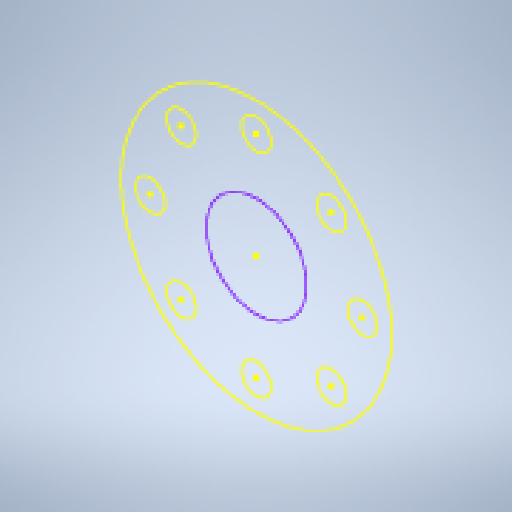
# Autodesk Inventor part: 부품69
Saved by Autodesk Inventor 2024 (Build 280153000, 153)
## iProperties
Created: 2024-09-08
Part Number: 부품69
Material: 일반
Document SubType Name: Modeling
Designer: Eungang
Density: 1 g/cm^3
Appearance: 기본값
Author: Eungang
Autodesk Inventor part; units mm, degrees
ref_plane "YZ Plane" through (0, 0, 0) normal (1, 0, 0) x (0, 1, 0)
ref_plane "XZ Plane" through (0, 0, 0) normal (0, 1, 0) x (-1, 0, 0)
ref_plane "XY Plane" through (0, 0, 0) normal (0, 0, 1) x (1, 0, 0)
sketch "스케치1" plane through (0, 0, 0) normal (0, 0, 1) x (1, 0, 0)
  circle A0 centre (-7.7782, -7.7782) radius 1.55 projected
  circle A1 centre (7.7782, -7.7782) radius 1.55 projected
  circle A2 centre (7.7782, 7.7782) radius 1.55 projected
  circle A3 centre (-7.7782, 7.7782) radius 1.55 projected
  circle A4 centre (0, 11) radius 1.55 projected
  circle A5 centre (11, 0) radius 1.55 projected
  circle A6 centre (0, -11) radius 1.55 projected
  circle A7 centre (-11, 0) radius 1.55 projected
  circle A8 centre (0, 0) radius 14 projected
  arc A9 (0, -5.2) -> (0, 5.2) centre (0, 0) ccw
  line L0 (32.5, -23) -> (32.5001, 127) projected
  line L1 (26.5, -23) -> (32.5, -23) projected
  line L2 (26.5001, 127) -> (26.5, -23) projected
  line L3 (32.5001, 127) -> (26.5001, 127) projected
  line L4 (0, 14) -> (32.5, 14)
  line L5 (32.5, 14) -> (32.5, -12.55)
  line L6 (0, -12.55) -> (0, 14)
  line L7 (0, -14) -> (32.5, -14)
  line L8 (32.5, -14) -> (32.5, -12.55)
  line L9 (0, 5.2) -> (-9.6, 5.2)
  line L10 (-9.6, -5.2) -> (0, -5.2)
  line L11 (0, -5.2) -> (0, 5.2)
  arc A10 (-11.2, -8.4) -> (-11.2, 8.4) centre (0, 0) ccw
  arc A11 (-11.2, 8.4) -> (-9.6, 5.2) centre (-9.6, 7.2) ccw
  arc A12 (-9.6, -5.2) -> (-11.2, -8.4) centre (-9.6, -7.2) ccw
  line L12 (26.5, 0) -> (32.5, 0)
  line L13 (32.5, 0) -> (32.5, -3)
  line L14 (32.5, -3) -> (26.5, -3)
  line L15 (26.5, -3) -> (26.5, 0)
  line L16 (32.5, 0) -> (26.5, 0)
  line L17 (26.5, 0) -> (26.5, 3)
  line L18 (26.5, 3) -> (32.5, 3)
  line L19 (32.5, 3) -> (32.5, 0)
  point P0 (0, 0)
  point P1 (-12.9985, -5.2)
  point P2 (-12.9985, 5.2)
  point P3 (-11.2, 8.4)
  dimension "d1" = 2
  dimension "d4" = 3
  dimension "d5" = 3
  constraints: 32 end point, 15 point on circle, 8 point on line, 6 parallel, 5 tangent, 4 centre point, 4 horizontal, 4 perpendicular, 1 coincident, 1 collinear, 1 equal radius
  measures "d1" radius of A11
  measures "d4" distance of L12.end L13.end
  measures "d5" distance of L16.end L17.end
extrude "돌출1" add sketch "스케치1" along normal blind 6 contours A4 L6 A8 A12 L10 A9 | A4 L6 L9 A11 A8 | L4 L2 L7 A8 | L4 L0 L18 L2 | L18 L0 L12 L2 | L2 L14 L0 L7 | L12 L0 L14 L2
sketch "스케치2" plane through (0, 0, 6) normal (0, 0, 1) x (1, 0, 0)
  arc A0 (-9.6, -5.2) -> (-11.2, -8.4) centre (-9.6, -7.2) ccw projected
  arc A1 (-11.2, -8.4) -> (0, -14) centre (0, 0) ccw projected
  line L0 (0, -14) -> (32.5, -14) projected
  line L1 (32.5, -14) -> (32.5, 14) projected
  line L2 (32.5, 14) -> (0, 14) projected
  arc A2 (0, 14) -> (-11.2, 8.4) centre (0, 0) ccw projected
  arc A3 (-11.2, 8.4) -> (-9.6, 5.2) centre (-9.6, 7.2) ccw projected
  line L3 (-9.6, 5.2) -> (0, 5.2) projected
  arc A4 (0, -5.2) -> (0, 5.2) centre (0, 0) ccw projected
  line L4 (0, -5.2) -> (-9.6, -5.2) projected
  circle A5 centre (0, -11) radius 1.55 projected
  circle A6 centre (-7.7782, 7.7782) radius 1.55 projected
  circle A7 centre (-7.7782, -7.7782) radius 1.55 projected
  circle A8 centre (7.7782, -7.7782) radius 1.55 projected
  circle A9 centre (7.7782, 7.7782) radius 1.55 projected
  circle A10 centre (11, 0) radius 1.55 projected
  circle A11 centre (0, 11) radius 1.55 projected
  line L5 (32.5, 14) -> (26.5, 14)
  line L6 (26.5, 14) -> (26.5, -14)
  line L7 (26.5, -14) -> (32.5, -14)
  line L8 (32.5, -14) -> (32.5, 14)
  line L9 (32.5, -14) -> (32.5, 14) projected
  line L10 (32.5, 0) -> (26.5, 0)
  line L11 (26.5, 0) -> (26.5, -3)
  line L12 (26.5, -3) -> (32.5, -3)
  line L13 (32.5, -3) -> (32.5, 0)
  line L14 (32.5, 0) -> (26.5, 0)
  line L15 (26.5, 0) -> (26.5, 3)
  line L16 (26.5, 3) -> (32.5, 3)
  line L17 (32.5, 3) -> (32.5, 0)
  point P0 (0, 0)
  point P1 (32.5, -3)
  dimension "d6" = 6
  dimension "d7" = 3
  dimension "d8" = 3
  constraints: 24 end point, 6 parallel, 3 horizontal, 3 perpendicular, 3 point on line, 1 midpoint
  measures "d6" distance of L7.end L6.end
  measures "d7" distance of L11.end L10.end
  measures "d8" distance of L14.end L15.end
extrude "돌출2" cut sketch "스케치2" against normal blind 6 contours L6 L12 L1 L0 | L6 L2 L1 L16
